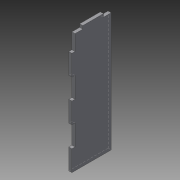
# Autodesk Inventor part: Motor support plate
Saved by Autodesk Inventor 2015 (Build 190159000, 159)
## iProperties
Created: 2014-11-12
Part Number: Motor support plate
Material: Generic
Document SubType Name: Modeling
Designer: karl
Density: 1 g/cm^3
Appearance: Default
Author: karl
Autodesk Inventor part; units mm, degrees
ref_plane "YZ Plane" through (0, 0, 0) normal (1, 0, 0) x (0, 1, 0)
ref_plane "XZ Plane" through (0, 0, 0) normal (0, 1, 0) x (-1, 0, 0)
ref_plane "XY Plane" through (0, 0, 0) normal (0, 0, 1) x (1, 0, 0)
sketch "Sketch1" plane through (0, 0, 0) normal (1, 0, 0) x (0, 1, 0)
  line L0 (-17.5, 57.5) -> (17.5, 57.5)
  line L1 (17.5, 57.5) -> (17.5, -57.5)
  line L2 (17.5, -57.5) -> (-17.5, -57.5)
  line L3 (-17.5, -57.5) -> (-17.5, 57.5)
  line L4 (-17.5, 57.5) -> (17.5, -57.5) construction
  line L5 (17.5, 57.5) -> (-17.5, -57.5) construction
  point P0 (0, 0)
  dimension "d0" = 35
  dimension "d1" = 115
  constraints: 12 end point, 2 midpoint, 2 parallel, 1 horizontal, 1 perpendicular
  measures "d0" distance of L1.end L2.end
  measures "d1" distance of L0.end L1.end
extrude "Extrusion1" add sketch "Sketch1" along normal blind 3
sketch "Sketch2" plane through (3, 0, 0) normal (1, 0, 0) x (0, 0, -1)
  line L0 (-57.5, -17.5) -> (57.5, -17.5) projected
  line L1 (-42.5, -17.5) -> (-22.5, -17.5)
  line L2 (-22.5, -17.5) -> (-22.5, -20.5)
  line L3 (-22.5, -20.5) -> (-42.5, -20.5)
  line L4 (-42.5, -20.5) -> (-42.5, -17.5)
  line L5 (-57.5, 17.5) -> (-57.5, -17.5) projected
  line L6 (-2.5, -17.5) -> (17.5, -17.5)
  line L7 (17.5, -17.5) -> (17.5, -20.5)
  line L8 (17.5, -20.5) -> (-2.5, -20.5)
  line L9 (-2.5, -20.5) -> (-2.5, -17.5)
  line L10 (37.5, -17.5) -> (57.5, -17.5)
  line L11 (57.5, -17.5) -> (57.5, -20.5)
  line L12 (57.5, -20.5) -> (37.5, -20.5)
  line L13 (37.5, -20.5) -> (37.5, -17.5)
  point P0 (0, 0)
  dimension "d4" = 20
  dimension "d5" = 3
  dimension "d6" = 15
  dimension "d7" = 20
  dimension "d8" = 3
  dimension "d9" = 20
  dimension "d10" = 20
  dimension "d11" = 3
  dimension "d12" = 20
  constraints: 24 end point, 6 parallel, 3 horizontal, 3 perpendicular, 3 point on line
  measures "d4" distance of L2.end L3.end
  measures "d5" distance of L1.end L2.end
  measures "d6" distance between parallel lines of L5 L4
  measures "d7" distance of L7.end L8.end
  measures "d8" distance of L6.end L7.end
  measures "d9" distance between parallel lines of L9 L2
  measures "d10" distance of L11.end L12.end
  measures "d11" distance of L10.end L11.end
  measures "d12" distance between parallel lines of L13 L7
extrude "Extrusion2" add sketch "Sketch2" against normal blind 3
sketch "Sketch3" plane through (3, 0, 0) normal (1, 0, 0) x (0, 0, -1)
  line L0 (-57.5, -17.5) -> (-57.5, 17.5) projected
  line L1 (-57.5, 10) -> (-60.5, 10)
  line L2 (-60.5, 10) -> (-60.5, -10)
  line L3 (-60.5, -10) -> (-57.5, -10)
  line L4 (-57.5, -10) -> (-57.5, 10)
  point P0 (0, 0)
  point P1 (-60.5, 0)
  dimension "d15" = 3
  dimension "d16" = 20
  constraints: 8 end point, 2 parallel, 1 horizontal, 1 horizontal alignment, 1 midpoint, 1 perpendicular, 1 point on line
  measures "d15" distance of L3.end L2.end
  measures "d16" distance of L2.end L1.end
extrude "Extrusion3" add sketch "Sketch3" against normal blind 3
sketch "Sketch4" plane through (3, 0, 0) normal (1, 0, 0) x (0, 0, -1)
  line L0 (-26.5, -7.5) -> (-14.5, -7.5)
  line L1 (-14.5, -7.5) -> (-14.5, 2.5)
  line L2 (-14.5, 2.5) -> (-26.5, 2.5)
  line L3 (-26.5, 2.5) -> (-26.5, -7.5)
  line L4 (-26.5, -7.5) -> (-14.5, 2.5) construction
  line L5 (-14.5, -7.5) -> (-26.5, 2.5) construction
  circle A0 centre (-20.5, -2.5) radius 2 projected
  point P0 (0, 0)
  point P1 (-20.5, -2.5)
  dimension "d19" = 12
  dimension "d20" = 10
  constraints: 12 end point, 3 midpoint, 2 parallel, 1 coincident, 1 horizontal, 1 perpendicular
  measures "d19" distance of L2.end L1.end
  measures "d20" distance of L1.end L0.end
extrude "Extrusion4" cut sketch "Sketch4" against normal blind 3 contours L3 L2 L1 L0 | A0
body "Solid1"
